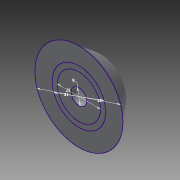
# Autodesk Inventor part: boltCap
Saved by Autodesk Inventor 2014 SP2 (Build 180246200, 246)
## iProperties
Created: 2019-05-11
Part Number: boltCap
Material: Generic
Document SubType Name: Modeling
Designer: GauchoHP
Density: 1 g/cm^3
Appearance: Default
Author: GauchoHP
Autodesk Inventor part; units mm, degrees
ref_plane "YZ Plane" through (0, 0, 0) normal (1, 0, 0) x (0, 1, 0)
ref_plane "XZ Plane" through (0, 0, 0) normal (0, 1, 0) x (-1, 0, 0)
ref_plane "XY Plane" through (0, 0, 0) normal (0, 0, 1) x (1, 0, 0)
sketch "Sketch1" plane through (0, 0, 0) normal (0, 1, 0) x (-1, 0, 0)
  circle A0 centre (0, 0) radius 12.5
  circle A1 centre (0, 0) radius 15.5
  circle A2 centre (0, 0) radius 25.5
  circle A3 centre (0, 0) radius 4.5
  dimension "d0" = 25
  dimension "d1" = 31
  dimension "d2" = 51
  dimension "d3" = 9
  constraints: 4 centre point, 4 coincident
  measures "d0" diameter of A0
  measures "d1" diameter of A1
  measures "d2" diameter of A2
  measures "d3" diameter of A3
extrude "Extrusion1" add sketch "Sketch1" along normal blind 3 contours A0 | A1 | A2
chamfer "Chamfer1" distance 3 angle 45 1 edges at (25.5, 3, 0)
extrude "Extrusion2" add sketch "Sketch1" along normal blind 13 contours A1
chamfer "Chamfer2" distance 7 distance2 9 1 edges at (15.5, 3, 0) measured on face at (-19.7987, 3, -3.0313)
fillet "Fillet1" radius 2 2 edges at (15.5, 13, 0) (12.5, 13, 0)
body "Solid1"
